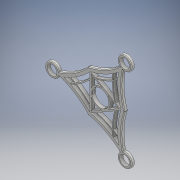
# Autodesk Inventor part: TriForce Pour Tri
Saved by Autodesk Inventor 2017 (Build 210142000, 142)
## iProperties
Part Number: TriForce Pour Tri
Material: Générique
Document SubType Name: Modeling
Designer: Thomas
Density: 1 g/cm^3
Appearance: Par défaut
Author: Thomas
Autodesk Inventor part; units mm, degrees
ref_plane "YZ Plane" through (0, 0, 0) normal (1, 0, 0) x (0, 1, 0)
ref_plane "XZ Plane" through (0, 0, 0) normal (0, 1, 0) x (-1, 0, 0)
sketch "Esquisse1" plane through (0, 0, 0) normal (0, 1, 0) x (-1, 0, 0)
  line L0 (0, 0) -> (-34.5, 59.755753) construction
  line L1 (0, 0) -> (-34.5, -59.755753) construction
  line L2 (0, 0) -> (69, 0) construction
  line L3 (17.25, 29.877876) -> (17.038476, 30)
  arc A0 (59.346819, -2.610764) -> (59.346819, 2.610764) centre (69, 0) ccw
  arc A1 (-31.93439, -50.090472) -> (-27.412427, -52.701229) centre (-34.5, -59.755753) ccw
  arc A2 (-27.412427, 52.701229) -> (-31.93439, 50.090472) centre (-34.5, 59.755753) ccw
  line L4 (17.038476, 30) -> (17.25, -29.877876) construction
  line L5 (-34.5, 0) -> (17.25, -29.877876) construction
  line L6 (17.038476, 30) -> (-34.5, 0) construction
  arc A3 (59.346819, -2.610764) -> (17.25, -29.877876) centre (89.659506, -95.539067) ccw
  arc A4 (17.25, 29.877876) -> (59.346819, 2.610764) centre (89.659506, 95.539067) ccw
  line L7 (69, 0) -> (60.339746, 5) construction
  line L8 (17.25, 29.877876) -> (17.038476, 30) construction
  arc A5 (-27.412427, 52.701229) -> (17.25, 29.877876) centre (37.909365, 125.416699) ccw
  arc A6 (-34.5, 0) -> (-31.93439, 50.090472) centre (-127.56873, 29.877876) ccw
  arc A7 (17.25, -29.877876) -> (-27.412427, -52.701229) centre (37.909365, -125.416699) ccw
  arc A8 (-31.93439, -50.090472) -> (-34.5, 0) centre (-127.56873, -29.877876) ccw
  circle A9 centre (69, 0) radius 7
  circle A10 centre (-34.5, 59.755753) radius 7
  circle A11 centre (-34.5, -59.755753) radius 7
  dimension "d0" = 69
  dimension "d1" = 69
  dimension "d2" = 69
  dimension "d3" = 120
  dimension "d4" = 120
  dimension "d5" = 20
  dimension "d6" = 20
  dimension "d7" = 20
  dimension "d9" = 60
  dimension "d10" = 97.74727
  dimension "d11" = 97.747
  dimension "d12" = 97.747
  dimension "d16" = 360
  constraints: 19 point on circle, 18 end point, 12 centre point, 4 coincident, 4 symmetric about line, 1 horizontal, 10 other
  measures "d0" distance of L0.start L0.end
  measures "d1" distance of L0.start L1.end
  measures "d2" distance of L0.start L2.end
  measures "d3" angle of L2 L0
  measures "d4" angle of L1 L2
  measures "d5" diameter of A0
  measures "d6" diameter of A1
  measures "d7" diameter of A2
  measures "d9" distance of L3.end L7.start
  measures "d10" radius of A3
  measures "d11" radius of A5
  measures "d12" radius of A7
sketch "Esquisse2" plane through (0, 0, 0) normal (0, 1, 0) x (-1, 0, 0)
  line L0 (12.049125, -20.90633) -> (11.900987, 21.028416)
  line L1 (11.900987, 21.028416) -> (-24.193361, 0.018279)
  line L2 (-24.193361, 0.018279) -> (12.049125, -20.90633)
  circle A0 centre (0, 0) radius 12.080906
  constraints: 6 end point, 1 centre point, 1 coincident
extrude "Extrusion1" add sketch "Esquisse1" along normal blind 5
extrude "Extrusion2" cut sketch "Esquisse2" along normal blind 5 contours L2 A0 L0 | A0 L0 | L2 L1 L0 A0 picked at (-0.213597, 5.744974)
fillet "Congé1" radius 1 27 edges at (-79, 5, 0) (-79, 0, 0) (-36.5197, 5, -13.4983) (-36.5197, 5, 13.4983) (-36.5197, 0, 13.4983) (6.57, 5, 38.3761) (-17.25, 2.5, 29.8779) (6.57, 0, 38.3761) (39.5, 5, 68.416) (39.5, 0, 68.416) (29.9497, 0, 24.8779) (34.5, 2.5, 0) (29.9497, 5, 24.8779) (29.9497, 5, -24.8779) (29.9497, 0, -24.8779) (39.5, 0, -68.416) (39.5, 5, -68.416) (6.57, 5, -38.3761) (6.0721, 0, -10.444) (-11.9751, 0, 0.061) (-11.9751, 5, 0.061) (6.0721, 5, -10.444) (6.1462, 5, 10.5233) (-36.5197, 0, -13.4983) (6.57, 0, -38.3761) (-17.25, 2.5, -29.8779) (6.1462, 0, 10.5233)
sketch "Esquisse3" plane through (0, 5, 0) normal (0, 1, 0) x (1, 0, 0)
  arc A0 (33.450281, 0) -> (31.19244, -51.385565) centre (127.56873, -29.877876) ccw
  arc A1 (31.19244, 51.385565) -> (33.450281, 0) centre (127.56873, 29.877876) ccw
  arc A2 (31.19244, 51.385565) -> (28.904985, 52.706228) centre (34.5, 59.755753) ccw
  arc A3 (-16.725141, 28.968793) -> (28.904985, 52.706228) centre (-37.909365, 125.416699) ccw
  arc A4 (-60.097426, 1.320669) -> (-16.725141, 28.968793) centre (-89.659506, 95.539067) ccw
  arc A5 (-60.097426, 1.320669) -> (-60.097426, -1.320669) centre (-69, 0) ccw
  arc A6 (-16.725141, -28.968793) -> (-60.097426, -1.320669) centre (-89.659506, -95.539067) ccw
  arc A7 (28.904985, -52.706228) -> (-16.725141, -28.968793) centre (-37.909365, -125.416699) ccw
  arc A8 (28.904985, -52.706228) -> (31.19244, -51.385565) centre (34.5, -59.755753) ccw
  circle A9 centre (34.5, 59.755753) radius 7
  circle A10 centre (34.5, -59.755753) radius 7
  circle A11 centre (-69, 0) radius 7
  line L0 (26.187236, -0.014743) -> (-13.055263, 22.641925)
  line L1 (-12.894862, -22.764018) -> (26.187236, -0.014743)
  line L2 (-13.055263, 22.641925) -> (-12.894862, -22.764018)
  line L3 (-54.396312, 0) -> (-19, 0) construction
  arc A12 (-35.194494, 0.800804) -> (-15.091197, 16.815889) centre (-88.659506, 88.539067) ccw
  arc A13 (-14.971957, -16.938401) -> (-35.194494, -0.800804) centre (-88.659506, -88.539067) ccw
  arc A14 (-36.531357, 0) -> (-43.497608, 3.748057) centre (-88.659506, -88.539067) ccw
  arc A15 (-14.9791, -14.916282) -> (-33.868967, 0) centre (-87.659506, -87.539067) ccw
  arc A16 (-35.194494, 0.800804) -> (-42.0135, 4.509575) centre (-87.659506, -87.539067) ccw
  arc A17 (-43.497608, -3.748057) -> (-36.531357, 0) centre (-88.659506, 88.539067) ccw
  arc A18 (-42.0135, -4.509575) -> (-35.194494, -0.800804) centre (-87.659506, 87.539067) ccw
  arc A19 (-33.868967, 0) -> (-15.084116, 14.811335) centre (-87.659506, 87.539067) ccw
  arc A20 (-13.035033, 16.915428) -> (-12.943435, 17.012342) centre (-87.659506, 87.539067) ccw
  line L4 (-14.971957, -16.938401) -> (-14.943435, -25.012342)
  line L5 (-15.119495, 24.826289) -> (-15.091197, 16.815889)
  line L6 (-15.084116, 14.811335) -> (-14.9791, -14.916282)
  arc A21 (24.994717, -35.796005) -> (18.265679, -31.637083) centre (-32.347328, -121.050918) ccw
  arc A22 (18.265679, -31.637083) -> (18.502891, -39.544062) centre (121.006834, -32.511851) ccw
  arc A23 (16.90373, -30.879728) -> (17.101344, -38.639546) centre (119.640809, -32.145826) ccw
  arc A24 (24.912157, -34.129971) -> (18.290764, -30.078924) centre (-31.981303, -119.684892) ccw
  arc A25 (22.155064, -4.496895) -> (18.290764, -30.078924) centre (121.006834, -32.511851) ccw
  arc A26 (20.407429, -5.51414) -> (16.934484, -29.331386) centre (119.640809, -32.145826) ccw
  arc A27 (16.934484, -29.331386) -> (-5.284934, -20.468895) centre (-31.981303, -119.684892) ccw
  arc A28 (16.90373, -30.879728) -> (-7.017389, -21.477305) centre (-32.347328, -121.050918) ccw
  arc A29 (18.502891, 39.544062) -> (18.265679, 31.637083) centre (121.006834, 32.511851) ccw
  arc A30 (18.265679, 31.637083) -> (24.994717, 35.796005) centre (-32.347328, 121.050918) ccw
  arc A31 (18.290764, 30.078924) -> (24.912157, 34.129971) centre (-31.981303, 119.684892) ccw
  arc A32 (17.101344, 38.639546) -> (16.90373, 30.879728) centre (119.640809, 32.145826) ccw
  arc A33 (-7.183107, 21.435295) -> (16.90373, 30.879728) centre (-32.347328, 121.050918) ccw
  arc A34 (-5.428329, 20.430422) -> (16.934484, 29.331386) centre (-31.981303, 119.684892) ccw
  arc A35 (16.934484, 29.331386) -> (20.36905, 5.65756) centre (119.640809, 32.145826) ccw
  arc A36 (18.290764, 30.078924) -> (22.108586, 4.661415) centre (121.006834, 32.511851) ccw
  line L7 (-13.642762, -25.578895) -> (-6.725003, -21.552141)
  line L8 (-4.997621, -20.54665) -> (20.330199, -5.803594)
  line L9 (22.072653, -4.78933) -> (29.045136, -0.730722)
  arc A37 (25.930023, -44.912118) -> (18.50289, -39.544046) centre (-37.909365, -125.416699) ccw
  arc A38 (17.101343, -38.63953) -> (-13.642762, -25.578895) centre (-37.909365, -125.416699) ccw
  arc A39 (29.045136, -0.730722) -> (24.912143, -34.129962) centre (127.56873, -29.877876) ccw
  arc A40 (24.994703, -35.795996) -> (25.930023, -44.912118) centre (127.56873, -29.877876) ccw
  arc A41 (-14.943435, -25.012342) -> (-42.0135, -4.509575) centre (-89.659506, -95.539067) ccw
  arc A42 (-43.497608, -3.748057) -> (-51.860075, 0) centre (-89.659506, -95.539067) ccw
  arc A43 (-51.860075, 0) -> (-43.497608, 3.748057) centre (-89.659506, 95.539067) ccw
  arc A44 (-42.0135, 4.509575) -> (-15.119495, 24.826289) centre (-89.659506, 95.539067) ccw
  arc A45 (-13.915219, 25.513065) -> (17.101343, 38.63953) centre (-37.909365, 125.416699) ccw
  arc A46 (18.50289, 39.544046) -> (25.930023, 44.912118) centre (-37.909365, 125.416699) ccw
  arc A47 (25.930023, 44.912118) -> (24.994703, 35.795996) centre (127.56873, 29.877876) ccw
  arc A48 (24.912143, 34.129962) -> (29.052572, 0.705599) centre (127.56873, 29.877876) ccw
  line L10 (29.052572, 0.705599) -> (22.09069, 4.725044)
  line L11 (20.349694, 5.730208) -> (-5.212341, 20.488456)
  line L12 (-6.953337, 21.49362) -> (-13.915219, 25.513065)
  point P0 (0, 0)
  point P1 (-13.943435, -18.012342)
  point P2 (-12.943435, -17.012342)
  point P3 (-13.943435, 18.012342)
  dimension "d25" = 360
  constraints: 90 point on circle, 37 centre point, 20 end point, 4 symmetric about line, 3 point on line, 1 horizontal, 73 other
extrude "Extrusion3" cut sketch "Esquisse3" against normal blind 5 contours A16 A44 L5 A12 | L4 A41 A18 A13 | A17 A42 A43 A14 | A15 A19 L6 | A40 A37 A22 A21 | A23 A38 L7 A28 | A24 A25 L9 A39 | A26 A27 L8 | A46 A47 A30 A29 | A31 A48 L10 A36 | A32 A33 L12 A45 | A34 A35 L11
ref_plane "Plan de construction1" through (0, 5, 0) normal (0, 1, 0) x (1, 0, 0)
sketch "Esquisse4" plane through (0, 5, 0) normal (0, 1, 0) x (1, 0, 0)
  circle A0 centre (0, 0) radius 12.186733
  circle A1 centre (0, 0) radius 14.109326
  constraints: 2 centre point, 2 coincident
extrude "Extrusion4" add sketch "Esquisse4" against normal blind 5
